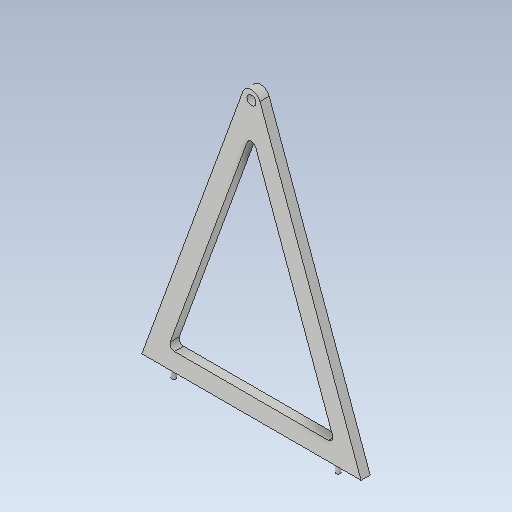
# Autodesk Inventor part: Outside
Saved by Autodesk Inventor 2020 (Build 240168000, 168)
## iProperties
Created: 2020-04-07
Part Number: Outside
Material: Generic
Document SubType Name: Modeling
Designer: gman
Density: 1 g/cm^3
Appearance: Default
Mass: 42.0846 g
Surface Area: 199.344 cm^2
Volume: 42.0846 cm^3
Author: gman
Autodesk Inventor part; units mm, degrees
ref_plane "YZ Plane" through (0, 0, 0) normal (1, 0, 0) x (0, 1, 0)
ref_plane "XZ Plane" through (0, 0, 0) normal (0, 1, 0) x (-1, 0, 0)
ref_plane "XY Plane" through (0, 0, 0) normal (0, 0, 1) x (1, 0, 0)
sketch "Sketch1" plane through (0, 0, 0) normal (0, 0, 1) x (1, 0, 0)
  circle A0 centre (0, 0) radius 3.175
  circle A1 centre (0, 0) radius 6.35
  line L0 (-5.967, 2.1718) -> (-76.0939, -190.5)
  line L1 (-76.0939, -190.5) -> (76.0939, -190.5)
  line L2 (76.0939, -190.5) -> (5.967, 2.1718)
  line L3 (0, -18.5662) -> (-57.9564, -177.8)
  line L4 (-57.9564, -177.8) -> (57.9564, -177.8)
  line L5 (57.9564, -177.8) -> (0, -18.5662)
  dimension "d0" = 6.35
  dimension "d1" = 12.7
  dimension "d2" = 70
  dimension "d3" = 70
  dimension "d4" = 190.5
  dimension "d5" = 12.7
  dimension "d9" = 152.1877
  constraints: 12 end point, 2 centre point, 2 coincident, 2 point on circle, 2 tangent, 1 horizontal
  measures "d0" diameter of A0
  measures "d1" diameter of A1
  measures "d2" angle of L1 L0
  measures "d3" angle of L1 L2
  measures "d4" distance from line of L1 point (0, 0)
  measures "d5" distance between parallel lines of L2 L5
  measures "d9" distance of L0.end L1.end
extrude "Extrusion1" add sketch "Sketch1" along normal blind 6.35
fillet "Fillet1" radius 3.175 3 edges at (0, -18.5662, 3.175) (-57.9564, -177.8, 3.175) (57.9564, -177.8, 3.175)
sketch "Sketch2" plane through (-76.0939, -190.5, 0) normal (0, -1, 0) x (1, 0, 0)
  circle A0 centre (19.05, 3.175) radius 1.5875
  circle A1 centre (133.1377, 3.175) radius 1.5875
  line L0 (0, 6.35) -> (152.1877, 6.35) projected
  line L1 (0, 0) -> (0, 6.35) projected
  line L2 (152.1877, 0) -> (152.1877, 6.35) projected
  point P0 (76.0939, 0)
  dimension "d10" = 3.175
  dimension "d11" = 3.175
  dimension "d12" = 19.05
  dimension "d13" = 19.05
  constraints: 2 centre point, 1 equal radius, 1 horizontal alignment
  measures "d10" diameter of A0
  measures "d11" distance from line of L0 A0.centre
  measures "d12" distance from line of L1 A0.centre
  measures "d13" distance from line of L2 A1.centre
extrude "Extrusion2" add sketch "Sketch2" along normal blind 6.35
body "Solid1"
